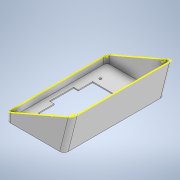
# Autodesk Inventor part: Front
Saved by Autodesk Inventor 2022 (Build 260153000, 153)
## iProperties
Created: 2021-06-27
Part Number: Front
Material: Generic
Document SubType Name: Modeling
Designer: Anton
Density: 1 g/cm^3
Appearance: Default
Author: Anton
Autodesk Inventor part; units mm, degrees
ref_plane "YZ Plane" through (0, 0, 0) normal (1, 0, 0) x (0, 1, 0)
ref_plane "XZ Plane" through (0, 0, 0) normal (0, 1, 0) x (-1, 0, 0)
sketch "Sketch1" plane through (0, 0, 0) normal (0, 1, 0) x (-1, 0, 0)
  line L0 (8, 0) -> (102.94, 0)
  line L1 (110.94, -8) -> (110.94, -185.2)
  line L2 (102.94, -193.2) -> (8, -193.2)
  line L3 (0, -185.2) -> (0, -8)
  circle A0 centre (86.7029, -32) radius 2.1
  circle A1 centre (88.297, -158.2) radius 2.1
  circle A2 centre (22.6, -158.501) radius 2.1
  circle A3 centre (21.4029, -32) radius 2.1
  arc A4 (110.94, -8) -> (102.94, 0) centre (102.94, -8) ccw
  arc A5 (8, 0) -> (0, -8) centre (8, -8) ccw
  arc A6 (0, -185.2) -> (8, -193.2) centre (8, -185.2) ccw
  arc A7 (102.94, -193.2) -> (110.94, -185.2) centre (102.94, -185.2) ccw
  point P0 (0, 0)
  dimension "d0" = 110.94
  dimension "d1" = 193.2
  dimension "d2" = 4.2
  dimension "d3" = 4.2
  dimension "d4" = 65.3
  dimension "d5" = 65.697
  dimension "d6" = 4.2
  dimension "d7" = 4.2
  dimension "d8" = 126.2
  dimension "d9" = 126.501
  dimension "d10" = 0
  dimension "d11" = 22.6
  dimension "d12" = 35
  dimension "d13" = 8
  constraints: 8 centre point, 8 end point, 8 point on circle, 8 tangent, 3 equal radius, 2 parallel, 2 point on line, 1 horizontal, 1 perpendicular
  measures "d0" distance between parallel lines of L3 L1
  measures "d1" distance between parallel lines of L2 L0
  measures "d2" diameter of A0
  measures "d3" diameter of A3
  measures "d4" distance of A3.centre A0.centre
  measures "d5" horizontal distance of A2.centre A1.centre
  measures "d6" diameter of A1
  measures "d7" diameter of A2
  measures "d8" vertical distance of A1.centre A0.centre
  measures "d9" vertical distance of A2.centre A3.centre
  measures "d10" vertical distance of A0.centre A3.centre
  measures "d11" distance from line of L3 A2.centre
  measures "d12" distance from line of L2 A1.centre
  measures "d13" radius of A4
extrude "Extrusion1" add sketch "Sketch1" along normal blind 2
sketch "Sketch3" plane through (0, 2, 0) normal (0, 1, 0) x (1, 0, 0)
  line L0 (-91, 41) -> (-12, 41)
  line L1 (-12, 41) -> (-12, 146)
  line L2 (-12, 146) -> (-91, 146)
  line L3 (-99.94, 72) -> (-91, 72)
  line L4 (-91, 118.2) -> (-99.94, 118.2)
  line L5 (-99.94, 118.2) -> (-99.94, 72)
  circle A0 centre (-88.297, 158.2) radius 2.1 projected
  circle A1 centre (-86.7029, 32) radius 2.1 projected
  line L6 (-91, 146) -> (-91, 118.2)
  line L7 (-91, 72) -> (-91, 41)
  line L8 (-102.94, 0) -> (-8, 0) projected
  line L9 (0, 8) -> (0, 185.2) projected
  line L10 (-110.94, 185.2) -> (-110.94, 8) projected
  point P0 (0, 0)
  dimension "d22" = 105
  dimension "d26" = 40
  dimension "d27" = 40
  dimension "d32" = 12
  dimension "d33" = 41
  dimension "d34" = 11
  dimension "d35" = 79
  dimension "d36" = 79
  constraints: 16 end point, 4 parallel, 2 horizontal, 1 perpendicular
  measures "d22" distance between parallel lines of L2 L0
  measures "d26" distance from line of L4 A0.centre
  measures "d27" distance from line of L3 A1.centre
  measures "d32" distance between parallel lines of L9 L1
  measures "d33" distance between parallel lines of L8 L0
  measures "d34" distance between parallel lines of L10 L5
  measures "d35" distance between parallel lines of L1 L6
  measures "d36" distance between parallel lines of L1 L7
extrude "Extrusion3" cut sketch "Sketch3" against normal blind 7.5 contours L7 L3 L5 L4 L6 L2 L1 L0
sketch "Sketch4" plane through (0, 2, 0) normal (0, 1, 0) x (1, 0, 0)
  line L0 (-91, 146) -> (-12, 146) projected
  line L1 (-12, 146) -> (-12, 41) projected
  line L2 (-12, 41) -> (-91, 41) projected
  line L3 (-91, 41) -> (-91, 72) projected
  line L4 (-91, 72) -> (-99.94, 72) projected
  line L5 (-99.94, 72) -> (-99.94, 118.2) projected
  line L6 (-99.94, 118.2) -> (-91, 118.2) projected
  line L7 (-91, 118.2) -> (-91, 146) projected
  line L8 (-8, 193.2) -> (-102.94, 193.2) projected
  arc A0 (-102.94, 193.2) -> (-110.94, 185.2) centre (-102.94, 185.2) ccw projected
  line L9 (-110.94, 185.2) -> (-110.94, 8) projected
  arc A1 (-110.94, 8) -> (-102.94, 0) centre (-102.94, 8) ccw projected
  line L10 (-102.94, 0) -> (-8, 0) projected
  arc A2 (-8, 0) -> (0, 8) centre (-8, 8) ccw projected
  line L11 (0, 8) -> (0, 185.2) projected
  arc A3 (0, 185.2) -> (-8, 193.2) centre (-8, 185.2) ccw projected
  circle A4 centre (-86.7029, 32) radius 2.1 projected
  circle A5 centre (-88.297, 158.2) radius 2.1 projected
  circle A6 centre (-22.6, 158.501) radius 2.1 projected
  circle A7 centre (-21.4029, 32) radius 2.1 projected
  arc A8 (-108.94, 8) -> (-102.94, 2) centre (-102.94, 8) ccw
  line L12 (-108.94, 8) -> (-108.94, 185.2)
  arc A9 (-102.94, 191.2) -> (-108.94, 185.2) centre (-102.94, 185.2) ccw
  line L13 (-102.94, 191.2) -> (-8, 191.2)
  arc A10 (-2, 185.2) -> (-8, 191.2) centre (-8, 185.2) ccw
  line L14 (-2, 185.2) -> (-2, 8)
  arc A11 (-8, 2) -> (-2, 8) centre (-8, 8) ccw
  line L15 (-8, 2) -> (-102.94, 2)
  point P0 (0, 0)
  dimension "d37" = 2
  constraints: 8 end point, 8 point on circle, 4 centre point, 7 other
  measures "d37" radial gap between concentric circles of A1 A8
extrude "Extrusion4" add sketch "Sketch4" along normal blind 60 contours A3 L11 A2 L10 A1 L9 A0 L8
sketch "Sketch5" plane through (-102.94, 0, 0) normal (0, 0, 1) x (1, 0, 0)
  line L0 (-8, 0) -> (-8, 62) projected
  line L1 (-8, 14) -> (102.94, 62)
  line L2 (102.94, 0) -> (102.94, 62) projected
  line L3 (0, 0) -> (-8, 0) projected
  line L4 (0, 62) -> (-8, 62) projected
  line L5 (-8, 14) -> (-8, 62)
  line L6 (102.94, 62) -> (94.94, 62) projected
  line L7 (-8, 62) -> (102.94, 62)
  dimension "d40" = 14
  dimension "d41" = 0
  constraints: 6 end point, 2 point on line, 1 perpendicular, 1 vertical
  measures "d40" distance from line of L3 L1.start
  measures "d41" distance of L2.end L1.end
extrude "Extrusion5" cut sketch "Sketch5" along normal mid plane 1000
sketch "Sketch6" plane through (-8, 0, -193.2) normal (0, 0, -1) x (-1, 0, 0)
  line L0 (102.94, 0) -> (102.94, 14) projected
  line L1 (102.94, 14) -> (-25.549, 69.5929)
  line L2 (94.94, 17.4613) -> (102.94, 14) projected
  line L3 (-25.549, 69.5929) -> (-8, 0)
  line L4 (0, 0) -> (-8, 0) projected
  line L5 (-8, 0) -> (0, 0)
  line L6 (0, 0) -> (0, 58.5387) projected
  line L7 (0, 0) -> (0, 58.5387)
  point P0 (-8, 62)
  dimension "d47" = 140
  constraints: 8 end point, 1 collinear, 1 horizontal, 1 point on line
  measures "d47" distance of L0.end L1.end
extrude "Extrusion6" add sketch "Sketch6" against normal blind 193.2
fillet "Fillet1" radius 8 2 edges at (8.7745, 34.7964, -193.2) (8.7745, 34.7964, 0)
ref_plane "Work Plane1" through (17.549, 69.5929, -193.2) normal (0.2445129, 0.9696461, 0) x (0, 0, 1)
sketch "Sketch9" plane through (17.549, 69.5929, -193.2) normal (0.2445129, 0.9696461, 0) x (0, 0, 1)
  line L0 (2, -22.0706) -> (191.2, -22.0706) projected
  line L1 (191.2, -100.3044) -> (191.2, -8.2462) projected
  line L2 (2, -22.0706) -> (191.2, -22.0706)
  line L3 (191.2, -22.0706) -> (191.2, -10)
  line L4 (183.2, -2) -> (10, -2)
  line L5 (2, -10) -> (2, -22.0706)
  line L6 (8, 0) -> (185.2, 0) projected
  arc A0 (191.2, -10) -> (183.2, -2) centre (183.2, -10) ccw
  arc A1 (10, -2) -> (2, -10) centre (10, -10) ccw
  point P0 (193.2, 0)
  point P1 (191.2, -2)
  dimension "d55" = 2
  dimension "d56" = 8
  constraints: 8 end point, 4 point on circle, 4 tangent, 3 point on line, 2 centre point, 2 parallel, 1 equal radius, 1 horizontal, 1 perpendicular
  measures "d55" distance between parallel lines of L6 L4
  measures "d56" radius of A0
extrude "Extrusion7" cut sketch "Sketch9" against normal up to surface surface through (-55.47, 2, -96.6) normal (0, 1, 0)
sketch "Sketch10" plane through (-110.94, 14, -8) normal (-0.397092, 0.9177788, 0) x (0.9177788, 0.397092, 0)
  line L0 (8.7167, -6) -> (127.3869, -6) projected
  ellipse E0 centre (8.7167, 0) end of major axis (15.2542, 0) minor radius 6 (2.1792, 0) -> (8.7167, -6) ccw projected
  line L1 (2.1792, 177.2) -> (2.1792, 0) projected
  ellipse E1 centre (8.7167, 177.2) end of major axis (15.2542, 177.2) minor radius 6 (8.7167, 183.2) -> (2.1792, 177.2) ccw projected
  line L2 (127.3869, 183.2) -> (8.7167, 183.2) projected
  ellipse E2 centre (127.3869, 175.2) end of major axis (137.4774, 175.2) minor radius 8 (137.4774, 175.2) -> (127.3869, 183.2) ccw projected
  line L3 (137.4774, 175.2) -> (137.4774, 2) projected
  ellipse E3 centre (127.3869, 2) end of major axis (117.2964, 2) minor radius 8 (127.3869, -6) -> (137.4774, 2) ccw projected
  ellipse E4 centre (129.9095, 0) end of major axis (140, 0) minor radius 8 (129.9095, -8) -> (140, 0) ccw projected
  line L4 (140, 177.2) -> (140, 0) projected
  ellipse E5 centre (129.9095, 177.2) end of major axis (140, 177.2) minor radius 8 (140, 177.2) -> (129.9095, 185.2) ccw projected
  line L5 (8.7167, 185.2) -> (129.9095, 185.2) projected
  ellipse E6 centre (8.7167, 177.2) end of major axis (0, 177.2) minor radius 8 (8.7167, 185.2) -> (0, 177.2) ccw projected
  line L6 (0, 0) -> (0, 177.2) projected
  ellipse E7 centre (8.7167, 0) end of major axis (0, 0) minor radius 8 (0, 0) -> (8.7167, -8) ccw projected
  line L7 (129.9095, -8) -> (8.7167, -8) projected
  point P0 (96.2591, -8)
  constraints: 8 other
body "Solid1"
